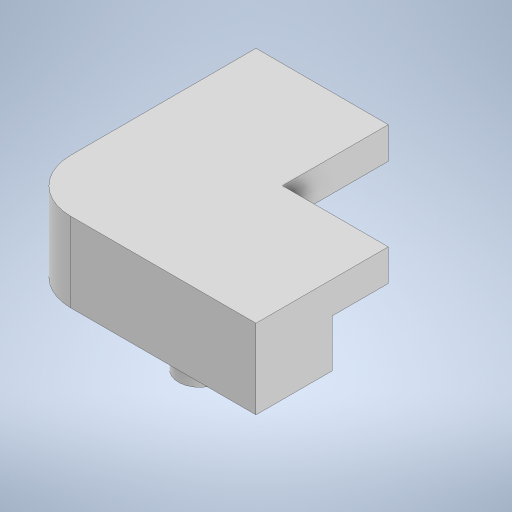
# Autodesk Inventor part: PresasPlaca_4
Saved by Autodesk Inventor 2023.2 (Build 272271030, 271C)
## iProperties
Created: 2023-01-18
Part Number: PresasPlaca_4
Material: Generic
Document SubType Name: Modeling
Designer: VICTOR
Density: 1 g/cm^3
Appearance: Default
Author: VICTOR
## iProperties of the stored document PresasPlaca_3DPrint.ipt
Created: 2023-04-30
Part Number: PresasPlaca_3DPrint
Material: Generic
Document SubType Name: Modeling
Designer: victo
Density: 1 g/cm^3
Appearance: Default
Author: victo
Autodesk Inventor part; units mm, degrees
ref_plane "YZ Plane" through (0, 0, 0) normal (1, 0, 0) x (0, 1, 0)
ref_plane "XZ Plane" through (0, 0, 0) normal (0, 1, 0) x (-1, 0, 0)
ref_plane "XY Plane" through (0, 0, 0) normal (0, 0, 1) x (1, 0, 0)
sketch "Sketch1" plane through (0, 0, 0) normal (0, 1, 0) x (-1, 0, 0)
  line L0 (0, 0) -> (10, 0)
  line L1 (0, 0) -> (20, 0)
  line L2 (20, 0) -> (20, -20)
  line L3 (20, -20) -> (0, -20)
  line L4 (0, -10) -> (0, 0)
  line L5 (10, -10) -> (10, -20)
  line L6 (10, -10) -> (0, -10)
  dimension "d3" = 20
  dimension "d4" = 20
  constraints: 14 end point, 2 horizontal, 2 parallel, 1 midpoint, 1 perpendicular
  measures "d3" distance of L2.end L3.end
  measures "d4" distance of L1.end L2.end
extrude "Extrusion1" add sketch "Sketch1" along normal blind 7.5
sketch "Sketch2" plane through (-10, 0, -10) normal (1, 0, 0) x (0, 0, -1)
  line L0 (0, 0) -> (10, 0) projected
  line L1 (10, 0) -> (10, 7.5) projected
  line L2 (0, 7.5) -> (10, 7.5) projected
  line L3 (0, 0) -> (0, 7.5) projected
  line L4 (-10, 0) -> (0, 0) projected
  line L5 (0, 0) -> (0, 7.5) projected
  line L6 (-10, 7.5) -> (0, 7.5) projected
  line L7 (-10, 0) -> (-10, 7.5) projected
  line L8 (10, 0) -> (10, 7.5) projected
  line L9 (10, 4.5) -> (-10, 4.5)
  point P0 (0, 4.5)
  dimension "d18" = 4.5
  constraints: 2 end point, 2 point on line, 1 perpendicular
  measures "d18" distance between parallel lines of L0 L9
extrude "Extrusion2" cut sketch "Sketch2" against normal blind 5.3 contours L3 L9 L1 L0
sketch "Sketch3" plane through (0, 7.5, -10) normal (0, 0, -1) x (-1, 0, 0)
  line L0 (0, -7.5) -> (15.3, -7.5) projected
  line L1 (15.3, -7.5) -> (15.3, -3) projected
  line L2 (10, -3) -> (15.3, -3) projected
  line L3 (10, -3) -> (10, 0) projected
  line L4 (0, 0) -> (10, 0) projected
  line L5 (0, -7.5) -> (0, 0) projected
  line L6 (10, -3) -> (0, -3)
  line L7 (0, -7.5) -> (0, 0) projected
  constraints: 2 end point, 1 horizontal, 1 point on line
extrude "Extrusion3" cut sketch "Sketch3" against normal blind 5.3 contours L5 L6 L2 L1 L0
sketch "Sketch4" plane through (0, 0, 0) normal (0, -1, 0) x (1, 0, 0)
  line L0 (-15.3, -20) -> (-15.3, -4.7) projected
  line L1 (-15.3, -4.7) -> (0, -4.7) projected
  line L2 (0, 0) -> (0, -4.7) projected
  line L3 (-20, 0) -> (0, 0) projected
  line L4 (-20, -20) -> (-20, 0) projected
  line L5 (-15.3, -20) -> (-20, -20) projected
  line L6 (0, 0) -> (0, -10) projected
  circle A0 centre (-10.33, -2.5) radius 2
  circle A1 centre (-17.5, -9.67) radius 2
  dimension "d11" = 4
  dimension "d12" = 4
  dimension "d16" = 9.67
  dimension "d17" = 9.67
  constraints: 2 centre point
  measures "d11" diameter of A0
  measures "d12" diameter of A1
  measures "d16" distance from line of L4 A0.centre
  measures "d17" distance from line of L3 A1.centre
extrude "Extrusion4" add sketch "Sketch4" along normal blind 4 contours A0 | A1
fillet "Fillet1" radius 2 1 edges at (-20, 3.75, 0)
sketch "Sketch5" plane through (0, 7.5, 0) normal (0, 1, 0) x (1, 0, 0)
  arc A0 (-20, 2) -> (-18, 0) centre (-18, 2) ccw projected
  line L0 (-18, 0) -> (0, 0) projected
  line L1 (0, 0) -> (0, 10) projected
  line L2 (0, 10) -> (-10, 10) projected
  line L3 (-10, 10) -> (-10, 20) projected
  line L4 (-10, 20) -> (-20, 20) projected
  line L5 (-20, 20) -> (-20, 2) projected
  line L6 (2.5, 22.5) -> (-22.5, 22.5)
  line L7 (-22.5, 22.5) -> (-22.5, -2.5)
  line L8 (-22.5, -2.5) -> (2.5, -2.5)
  line L9 (2.5, -2.5) -> (2.5, 22.5)
  line L10 (2.5, 22.5) -> (-22.5, -2.5) construction
  line L11 (-22.5, 22.5) -> (2.5, -2.5) construction
  line L12 (-15.3, 20) -> (-20, 20) projected
  line L13 (-20, 20) -> (-22.5, 20)
  line L14 (0, 0) -> (0, -2.5)
  dimension "d19" = 25
  dimension "d20" = 25
  constraints: 16 end point, 3 point on line, 2 midpoint, 2 parallel, 2 perpendicular, 1 horizontal
  measures "d19" distance of L8.end L7.end
  measures "d20" distance of L7.end L6.end
extrude "Extrusion5" add sketch "Sketch5" against normal blind 7.5 contours A0 L0 L14 L8 L7 L13 L5
fillet "Fillet2" radius 5 1 edges at (-22.5, 3.75, 2.5)
body "Solid1"
